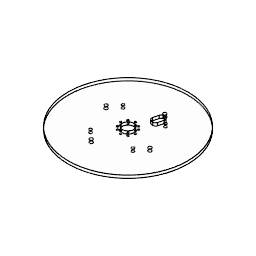
TopPlate_v60 (Autodesk Fusion 360 design; units mm, degrees)
Autodesk Fusion 360 part; units mm, degrees
note: some values were not read from the file. Set by a fixed rule: which face or edge a step refers to.
derive "Sketch1" from "ServoRail v52"
sketch "sketch 220" plane through (0, 0, 0) normal (0, 0, 1) x (1, 0, 0)
  line L0 (-23.75, 13.75) -> (23.75, 13.75) construction
  line L1 (23.75, 13.75) -> (23.75, -13.75) construction
  line L2 (23.75, -13.75) -> (-23.75, -13.75) construction
  line L3 (-23.75, -13.75) -> (-23.75, 13.75) construction
  line L4 (-23.75, 13.75) -> (23.75, -13.75) construction
  line L5 (23.75, 13.75) -> (-23.75, -13.75) construction
  line L6 (-2.75, -24.75) -> (-44.75, -24.75)
  line L7 (-44.75, -24.75) -> (-44.75, -2.75)
  line L8 (-44.75, -2.75) -> (-2.75, -2.75)
  line L9 (-2.75, -2.75) -> (-2.75, -24.75)
  line L10 (-2.75, -24.75) -> (-44.75, -2.75) construction
  line L11 (-44.75, -24.75) -> (-2.75, -2.75) construction
  line L12 (-32.75, -2.75) -> (-32.75, 4.25)
  line L13 (-32.75, 4.25) -> (-29.75, 4.25)
  line L14 (-29.75, 4.25) -> (-29.75, 0.25)
  line L15 (-26.75, 0.25) -> (-26.75, -2.75)
  line L16 (-26.75, 0.25) -> (-29.75, 0.25)
  line L17 (2.75, -44.75) -> (2.75, -2.75)
  line L18 (2.75, -32.75) -> (-4.25, -32.75)
  line L19 (-4.25, -32.75) -> (-4.25, -29.75)
  line L20 (-4.25, -29.75) -> (-0.25, -29.75)
  line L21 (-0.25, -26.75) -> (-0.25, -29.75)
  line L22 (-0.25, -26.75) -> (2.75, -26.75)
  line L23 (24.75, -44.75) -> (2.75, -44.75)
  line L24 (24.75, -2.75) -> (24.75, -44.75)
  line L25 (2.75, -2.75) -> (24.75, -2.75)
  line L26 (44.75, 2.75) -> (2.75, 2.75)
  line L27 (32.75, 2.75) -> (32.75, -4.25)
  line L28 (32.75, -4.25) -> (29.75, -4.25)
  line L29 (29.75, -4.25) -> (29.75, -0.25)
  line L30 (26.75, -0.25) -> (29.75, -0.25)
  line L31 (26.75, -0.25) -> (26.75, 2.75)
  line L32 (44.75, 24.75) -> (44.75, 2.75)
  line L33 (2.75, 24.75) -> (44.75, 24.75)
  line L34 (2.75, 2.75) -> (2.75, 24.75)
  line L35 (-2.75, 44.75) -> (-2.75, 2.75)
  line L36 (-2.75, 32.75) -> (4.25, 32.75)
  line L37 (4.25, 32.75) -> (4.25, 29.75)
  line L38 (4.25, 29.75) -> (0.25, 29.75)
  line L39 (0.25, 26.75) -> (0.25, 29.75)
  line L40 (0.25, 26.75) -> (-2.75, 26.75)
  line L41 (-24.75, 44.75) -> (-2.75, 44.75)
  line L42 (-24.75, 2.75) -> (-24.75, 44.75)
  line L43 (-2.75, 2.75) -> (-24.75, 2.75)
  line L44 (-0.25, -32.75) -> (-0.25, -35.75)
  line L45 (-0.25, -35.75) -> (-7.25, -35.75)
  line L46 (-7.25, -35.75) -> (-7.25, -26.75)
  line L47 (-7.25, -26.75) -> (-0.25, -26.75)
  line L48 (-26.75, -27.75) -> (-29.75, -27.75)
  line L49 (-29.75, -27.75) -> (-29.75, -24.75)
  line L50 (-26.75, -27.75) -> (-26.75, -31.75)
  line L51 (-26.75, -31.75) -> (-23.75, -31.75)
  line L52 (-23.75, -31.75) -> (-23.75, -24.75)
  line L53 (-29.75, -27.75) -> (-29.75, -34.75)
  line L54 (-29.75, -34.75) -> (-20.75, -34.75)
  line L55 (-20.75, -34.75) -> (-20.75, -27.75)
  line L56 (-20.75, -27.75) -> (-23.75, -27.75)
  line L57 (-20.75, -27.75) -> (-7.25, -27.75)
  line L58 (-20.75, -30.75) -> (-7.25, -30.75)
  line L59 (27.75, -29.75) -> (24.75, -29.75)
  line L60 (27.75, -29.75) -> (34.75, -29.75)
  line L61 (27.75, -26.75) -> (27.75, -29.75)
  line L62 (31.75, -23.75) -> (24.75, -23.75)
  line L63 (27.75, -26.75) -> (31.75, -26.75)
  line L64 (31.75, -26.75) -> (31.75, -23.75)
  line L65 (34.75, -29.75) -> (34.75, -20.75)
  line L66 (34.75, -20.75) -> (27.75, -20.75)
  line L67 (27.75, -20.75) -> (27.75, -23.75)
  line L68 (27.75, -20.75) -> (27.75, -7.25)
  line L69 (30.75, -20.75) -> (30.75, -7.25)
  line L70 (26.75, -7.25) -> (26.75, -0.25)
  line L71 (35.75, -7.25) -> (26.75, -7.25)
  line L72 (35.75, -0.25) -> (35.75, -7.25)
  line L73 (32.75, -0.25) -> (35.75, -0.25)
  line L74 (29.75, 27.75) -> (29.75, 24.75)
  line L75 (29.75, 27.75) -> (29.75, 34.75)
  line L76 (26.75, 27.75) -> (29.75, 27.75)
  line L77 (23.75, 31.75) -> (23.75, 24.75)
  line L78 (26.75, 27.75) -> (26.75, 31.75)
  line L79 (26.75, 31.75) -> (23.75, 31.75)
  line L80 (29.75, 34.75) -> (20.75, 34.75)
  line L81 (20.75, 34.75) -> (20.75, 27.75)
  line L82 (20.75, 27.75) -> (23.75, 27.75)
  line L83 (20.75, 27.75) -> (7.25, 27.75)
  line L84 (20.75, 30.75) -> (7.25, 30.75)
  line L85 (7.25, 26.75) -> (0.25, 26.75)
  line L86 (7.25, 35.75) -> (7.25, 26.75)
  line L87 (0.25, 35.75) -> (7.25, 35.75)
  line L88 (0.25, 32.75) -> (0.25, 35.75)
  line L89 (-27.75, 29.75) -> (-24.75, 29.75)
  line L90 (-27.75, 29.75) -> (-34.75, 29.75)
  line L91 (-27.75, 26.75) -> (-27.75, 29.75)
  line L92 (-31.75, 23.75) -> (-24.75, 23.75)
  line L93 (-27.75, 26.75) -> (-31.75, 26.75)
  line L94 (-31.75, 26.75) -> (-31.75, 23.75)
  line L95 (-34.75, 29.75) -> (-34.75, 20.75)
  line L96 (-34.75, 20.75) -> (-27.75, 20.75)
  line L97 (-27.75, 20.75) -> (-27.75, 23.75)
  line L98 (-27.75, 20.75) -> (-27.75, 7.25)
  line L99 (-30.75, 20.75) -> (-30.75, 7.25)
  line L100 (-26.75, 7.25) -> (-26.75, 0.25)
  line L101 (-35.75, 7.25) -> (-26.75, 7.25)
  line L102 (-35.75, 0.25) -> (-35.75, 7.25)
  line L103 (-32.75, 0.25) -> (-35.75, 0.25)
  circle A0 centre (0, 0) radius 56
  circle A1 centre (-41.3532, 14.4521) radius 9.125
  circle A2 centre (-14.4521, -41.3532) radius 9.125
  circle A3 centre (41.3532, -14.4521) radius 9.125
  circle A4 centre (14.4521, 41.3532) radius 9.125
  circle A5 centre (-41.3532, 14.4521) radius 11.125
  circle A6 centre (-14.4521, -41.3532) radius 11.125
  circle A7 centre (41.3532, -14.4521) radius 11.125
  circle A8 centre (14.4521, 41.3532) radius 11.125
  circle A9 centre (0, 0) radius 58
  line L104 (-41.3532, 14.4521) -> (-41.0042, 25.5716)
  line L105 (-41.3532, 14.4521) -> (-41.3532, 3.3271)
  line L106 (0, 0) -> (-41.3532, 14.4521) construction
  line L107 (-14.4521, -41.3532) -> (-25.5716, -41.0042)
  line L108 (-14.4521, -41.3532) -> (-3.3271, -41.3532)
  line L109 (41.3532, -14.4521) -> (41.0042, -25.5716)
  line L110 (41.3532, -14.4521) -> (41.3532, -3.3271)
  line L111 (14.4521, 41.3532) -> (25.5716, 41.0042)
  line L112 (14.4521, 41.3532) -> (3.3271, 41.3532)
  line L113 (2.75, 24.75) -> (-2.75, 24.75)
  line L114 (24.75, -2.75) -> (24.75, 2.75)
  line L115 (-24.75, 2.75) -> (-24.75, -2.75)
  line L116 (-2.75, -24.75) -> (2.75, -24.75)
  circle A10 centre (-7.9571, -31.4571) radius 1.75
  line L117 (-7.25, -30.75) -> (-7.9571, -31.4571)
  line L118 (-18.75, -31.75) -> (-22.75, -31.75)
  line L119 (-22.75, -31.75) -> (-22.75, -29.75)
  line L120 (-22.75, -29.75) -> (-18.75, -29.75)
  line L121 (-18.75, -29.75) -> (-18.75, -31.75)
  line L122 (-18.75, -31.75) -> (-22.75, -29.75) construction
  line L123 (-22.75, -31.75) -> (-18.75, -29.75) construction
  circle A11 centre (31.4571, -7.9571) radius 1.75
  line L124 (31.75, -22.75) -> (29.75, -22.75)
  line L125 (29.75, -22.75) -> (29.75, -18.75)
  line L126 (29.75, -18.75) -> (31.75, -18.75)
  line L127 (31.75, -18.75) -> (31.75, -22.75)
  circle A12 centre (7.9571, 31.4571) radius 1.75
  line L128 (22.75, 31.75) -> (22.75, 29.75)
  line L129 (22.75, 29.75) -> (18.75, 29.75)
  line L130 (18.75, 29.75) -> (18.75, 31.75)
  line L131 (18.75, 31.75) -> (22.75, 31.75)
  circle A13 centre (-31.4571, 7.9571) radius 1.75
  line L132 (-31.75, 22.75) -> (-29.75, 22.75)
  line L133 (-29.75, 22.75) -> (-29.75, 18.75)
  line L134 (-29.75, 18.75) -> (-31.75, 18.75)
  line L135 (-31.75, 18.75) -> (-31.75, 22.75)
  line L136 (29.75, 27.75) -> (33.8506, 28.3482) construction
  circle A14 centre (33.8506, 28.3482) radius 1.75
  circle A15 centre (-28.3482, 33.8506) radius 1.75
  circle A16 centre (-33.8506, -28.3482) radius 1.75
  circle A17 centre (28.3482, -33.8506) radius 1.75
  line L137 (-6.25, -7.75) -> (-14.25, -7.75)
  line L138 (-14.25, -7.75) -> (-14.25, -19.75)
  line L139 (-14.25, -19.75) -> (-6.25, -19.75)
  line L140 (-6.25, -19.75) -> (-6.25, -7.75)
  line L141 (-6.25, -7.75) -> (-14.25, -19.75) construction
  line L142 (-14.25, -7.75) -> (-6.25, -19.75) construction
  line L143 (19.75, -14.25) -> (19.75, -6.25)
  line L144 (7.75, -14.25) -> (19.75, -14.25)
  line L145 (19.75, -6.25) -> (7.75, -6.25)
  line L146 (7.75, -6.25) -> (7.75, -14.25)
  line L147 (14.25, 19.75) -> (6.25, 19.75)
  line L148 (14.25, 7.75) -> (14.25, 19.75)
  line L149 (6.25, 19.75) -> (6.25, 7.75)
  line L150 (6.25, 7.75) -> (14.25, 7.75)
  line L151 (-19.75, 14.25) -> (-19.75, 6.25)
  line L152 (-7.75, 14.25) -> (-19.75, 14.25)
  line L153 (-19.75, 6.25) -> (-7.75, 6.25)
  line L154 (-7.75, 6.25) -> (-7.75, 14.25)
  spline S0 degree 5 poles (-3.3271, -41.3532) (-3.3271, -42.1374) (-3.2169, -43.6541) (-2.7212, -45.7746) (-1.5233, -48.3293) (0.3412, -51.1793) (1.6763, -53.2302) (2.3663, -54.6364) (2.6513, -55.5109) (2.75, -55.9324) knots 0 0 0 0 0 0 0.2 0.4 0.6 0.8 1 1 1 1 1 1
  line L155 (-3.3271, -39.4276) -> (-3.3271, -43.2787)
  line L156 (2.5, -54.8649) -> (3, -57)
  line L157 (2.75, -44.75) -> (2.75, -55.9324) construction
  spline S1 degree 3 poles (-5.3271, -41.3532) (-5.3271, -43.6244) (-4.7917, -45.7291) (-3.9986, -47.5464) (-3.0648, -49.6861) (-1.8311, -51.476) (-0.8806, -52.9928) (-0.0937, -54.2485) (0.4782, -55.3083) (0.7178, -56.0783) (0.7516, -56.1872) (0.7797, -56.2904) (0.8027, -56.3885) knots 0 0 0 0 0.303965 0.303965 0.303965 0.661847 0.661847 0.661847 0.958125 0.958125 0.958125 1 1 1 1
  line L158 (0.6913, -55.9957) -> (2.75, -55.9324)
  spline S2 degree 5 poles (41.3532, -3.3271) (42.1374, -3.3271) (43.6541, -3.2169) (45.7746, -2.7212) (48.3293, -1.5233) (51.1793, 0.3412) (53.2302, 1.6763) (54.6364, 2.3663) (55.5109, 2.6513) (55.9324, 2.75) knots 0 0 0 0 0 0 0.2 0.4 0.6 0.8 1 1 1 1 1 1
  spline S3 degree 3 poles (41.3532, -5.3271) (43.6244, -5.3271) (45.7291, -4.7917) (47.5464, -3.9986) (49.6861, -3.0648) (51.476, -1.8311) (52.9928, -0.8806) (54.2485, -0.0937) (55.3083, 0.4782) (56.0783, 0.7178) (56.1872, 0.7516) (56.2904, 0.7797) (56.3885, 0.8027) knots 0 0 0 0 0.303965 0.303965 0.303965 0.661847 0.661847 0.661847 0.958125 0.958125 0.958125 1 1 1 1
  line L159 (55.9957, 0.6913) -> (55.9324, 2.75)
  spline S4 degree 5 poles (3.3271, 41.3532) (3.3271, 42.1374) (3.2169, 43.6541) (2.7212, 45.7746) (1.5233, 48.3293) (-0.3412, 51.1793) (-1.6763, 53.2302) (-2.3663, 54.6364) (-2.6513, 55.5109) (-2.75, 55.9324) knots 0 0 0 0 0 0 0.2 0.4 0.6 0.8 1 1 1 1 1 1
  spline S5 degree 3 poles (5.3271, 41.3532) (5.3271, 43.6244) (4.7917, 45.7291) (3.9986, 47.5464) (3.0648, 49.6861) (1.8311, 51.476) (0.8806, 52.9928) (0.0937, 54.2485) (-0.4782, 55.3083) (-0.7178, 56.0783) (-0.7516, 56.1872) (-0.7797, 56.2904) (-0.8027, 56.3885) knots 0 0 0 0 0.303965 0.303965 0.303965 0.661847 0.661847 0.661847 0.958125 0.958125 0.958125 1 1 1 1
  line L160 (-0.6913, 55.9957) -> (-2.75, 55.9324)
  spline S6 degree 5 poles (-41.3532, 3.3271) (-42.1374, 3.3271) (-43.6541, 3.2169) (-45.7746, 2.7212) (-48.3293, 1.5233) (-51.1793, -0.3412) (-53.2302, -1.6763) (-54.6364, -2.3663) (-55.5109, -2.6513) (-55.9324, -2.75) knots 0 0 0 0 0 0 0.2 0.4 0.6 0.8 1 1 1 1 1 1
  spline S7 degree 3 poles (-41.3532, 5.3271) (-43.6244, 5.3271) (-45.7291, 4.7917) (-47.5464, 3.9986) (-49.6861, 3.0648) (-51.476, 1.8311) (-52.9928, 0.8806) (-54.2485, 0.0937) (-55.3083, -0.4782) (-56.0783, -0.7178) (-56.1872, -0.7516) (-56.2904, -0.7797) (-56.3885, -0.8027) knots 0 0 0 0 0.303965 0.303965 0.303965 0.661847 0.661847 0.661847 0.958125 0.958125 0.958125 1 1 1 1
  line L161 (-55.9957, -0.6913) -> (-55.9324, -2.75)
  line L162 (-29.75, -34.75) -> (-37.9688, -34.75)
  line L163 (-29.75, -32.75) -> (-38, -32.75)
  spline S8 degree 5 poles (-37.9688, -34.75) (-38.3782, -34.75) (-39.1998, -34.6725) (-40.4402, -34.3239) (-42.1078, -33.4585) (-44.2076, -31.9324) (-45.8949, -30.4934) (-47.1632, -29.3318) (-48.0099, -28.5231) (-48.4336, -28.1103) knots 0 0 0 0 0 0 0.2 0.4 0.6 0.8 1 1 1 1 1 1
  line L164 (-37, -34.75) -> (-38.9375, -34.75)
  spline S9 degree 3 poles (-37.9688, -32.75) (-38.6389, -32.75) (-39.3828, -32.5469) (-40.2776, -32.0885) (-41.7597, -31.3293) (-43.513, -29.9305) (-45.2704, -28.34) (-45.8565, -27.8096) (-46.4464, -27.2542) (-47.0377, -26.678) knots 0 0 0 0 0.31167 0.31167 0.31167 0.827845 0.827845 0.827845 1 1 1 1
  line L165 (-48.4336, -28.1103) -> (-47.0377, -26.678)
  line L166 (34.75, -29.75) -> (34.75, -37.9688)
  line L167 (32.75, -29.75) -> (32.75, -38)
  spline S10 degree 3 poles (32.75, -37.9688) (32.75, -38.6389) (32.5469, -39.3828) (32.0885, -40.2776) (31.3293, -41.7597) (29.9305, -43.513) (28.34, -45.2704) (27.8096, -45.8565) (27.2542, -46.4464) (26.678, -47.0377) knots 0 0 0 0 0.31167 0.31167 0.31167 0.827845 0.827845 0.827845 1 1 1 1
  spline S11 degree 5 poles (34.75, -37.9688) (34.75, -38.3782) (34.6725, -39.1998) (34.3239, -40.4402) (33.4585, -42.1078) (31.9324, -44.2076) (30.4934, -45.8949) (29.3318, -47.1632) (28.5231, -48.0099) (28.1103, -48.4336) knots 0 0 0 0 0 0 0.2 0.4 0.6 0.8 1 1 1 1 1 1
  line L168 (28.1103, -48.4336) -> (26.678, -47.0377)
  line L169 (29.75, 34.75) -> (37.9688, 34.75)
  line L170 (29.75, 32.75) -> (38, 32.75)
  spline S12 degree 3 poles (37.9688, 32.75) (38.6389, 32.75) (39.3828, 32.5469) (40.2776, 32.0885) (41.7597, 31.3293) (43.513, 29.9305) (45.2704, 28.34) (45.8565, 27.8096) (46.4464, 27.2542) (47.0377, 26.678) knots 0 0 0 0 0.31167 0.31167 0.31167 0.827845 0.827845 0.827845 1 1 1 1
  spline S13 degree 5 poles (37.9688, 34.75) (38.3782, 34.75) (39.1998, 34.6725) (40.4402, 34.3239) (42.1078, 33.4585) (44.2076, 31.9324) (45.8949, 30.4934) (47.1632, 29.3318) (48.0099, 28.5231) (48.4336, 28.1103) knots 0 0 0 0 0 0 0.2 0.4 0.6 0.8 1 1 1 1 1 1
  line L171 (48.4336, 28.1103) -> (47.0377, 26.678)
  line L172 (-34.75, 29.75) -> (-34.75, 37.9688)
  line L173 (-32.75, 29.75) -> (-32.75, 38)
  spline S14 degree 3 poles (-32.75, 37.9688) (-32.75, 38.6389) (-32.5469, 39.3828) (-32.0885, 40.2776) (-31.3293, 41.7597) (-29.9305, 43.513) (-28.34, 45.2704) (-27.8096, 45.8565) (-27.2542, 46.4464) (-26.678, 47.0377) knots 0 0 0 0 0.31167 0.31167 0.31167 0.827845 0.827845 0.827845 1 1 1 1
  spline S15 degree 5 poles (-34.75, 37.9688) (-34.75, 38.3782) (-34.6725, 39.1998) (-34.3239, 40.4402) (-33.4585, 42.1078) (-31.9324, 44.2076) (-30.4934, 45.8949) (-29.3318, 47.1632) (-28.5231, 48.0099) (-28.1103, 48.4336) knots 0 0 0 0 0 0 0.2 0.4 0.6 0.8 1 1 1 1 1 1
  line L174 (-28.1103, 48.4336) -> (-26.678, 47.0377)
  point P0 (-23.75, -13.75)
  point P1 (-20.75, -30.75)
  point P2 (-10.25, -13.75)
extrude "Extrude1" add sketch "sketch 220" along normal blind 3 contours L6 L17 L22 L46 L47 L52 L56 L57 L116 | L6 L7 L8 L9 | L8 L9 L17 L25 L26 L34 L35 L43 L113 L114 L115 L116 | L6 L48 L49 L50 L51 L52 | L17 L23 L24 L25 | L6 L7 L8 L12 L49 L53 L102 L103 A0 A5 S6 L163 S9 L165 | L48 L50 L51 L52 L53 L54 L55 L56 A6 L118 L119 L120 | L8 L15 L42 L92 L97 L98 L100 L101 L115 | L17 L18 L19 L20 L21 L22 | L46 L55 L57 L58 A6 A10 L120 L121 | L8 L12 L13 L14 L15 L16 | L35 L41 L42 L43 | L17 L18 L23 L24 L44 L45 L59 L60 A0 A6 S0 L167 S10 L168 | L18 L19 L20 L21 L44 L45 L46 L47 A6 A10 | L24 L26 L31 L62 L67 L68 L70 L71 L114 | L53 L162 L163 S8 L164 S9 L165 | L55 L58 L120 L121 | L55 L118 L119 L120 | L12 L13 L14 L16 L100 L101 L102 L103 A5 A13 | L42 L89 L91 L92 L93 L94 | L24 L59 L61 L62 L63 L64 | L26 L32 L33 L34 | L54 A0 A6 S1 L162 S8 L164 | L55 L58 A6 L118 L121 | L35 L36 L41 L42 L87 L88 L89 L90 A0 A8 S4 L173 S14 L174 | L90 L91 L92 L93 L94 L95 L96 L97 A5 L132 L133 L135 | L33 L35 L40 L77 L82 L83 L85 L86 L113 | L60 L61 L62 L63 L64 L65 L66 L67 A7 L124 L125 L127 | L26 L27 L28 L29 L30 L31 | L54 L55 A6 | L54 A2 A6 L107 | L55 A6 L118 | L58 A6 L121 | L58 A6 A10 | L96 L98 L99 L101 A5 A13 L133 L134 | L35 L36 L37 L38 L39 L40 | L45 A2 A6 L108 | L45 L46 A6 A10 | L66 L68 L69 L71 A7 A11 L125 L126 | L26 L27 L32 L33 L72 L73 L74 L75 A0 A7 S2 L170 S12 L171 | L27 L28 L29 L30 L70 L71 L72 L73 A7 A11 | L46 L55 L58 A2 A6 A10 L118 L121 | A2 L107 L108 | A2 A6 L107 S1 | A6 L118 L121 | L58 A6 | L102 A1 A5 L105 | L101 L102 A5 A13 | L90 L172 L173 S14 S15 L174 | L96 L99 L133 L134 | L96 L132 L133 L135 | L36 L37 L38 L39 L85 L86 L87 L88 A8 A12 | L33 L74 L76 L77 L78 L79 | A6 S0 S1 L158 | A6 L108 S1 | L60 L166 L167 S10 S11 L168 | L66 L69 L125 L126 | L66 L124 L125 L127 | A2 L107 L108 | L96 L99 L101 A1 A5 A13 L134 L135 | A1 L104 L105 | A5 S6 S7 L161 | A5 L105 S7 | L95 A0 A5 S7 L172 S15 | L96 L99 A5 L134 L135 | L75 L76 L77 L78 L79 L80 L81 L82 A8 L128 L129 L131 | A0 L158 | L65 A0 A7 S3 L166 S11 | L66 L69 A7 L126 L127 | A0 L161 | A1 A5 L104 S7 | A1 L104 L105 | L99 A5 A13 | L95 L96 A5 | L95 A1 A5 L104 | L96 A5 L135 | L99 A5 L134 | L81 L83 L84 L86 A8 A12 L129 L130 | L65 L66 A7 | L65 A3 A7 L109 | L66 A7 L127 | L69 A7 L126 | L71 L72 A7 A11 | L69 A7 A11 | L72 A3 A7 L110 | L99 A5 | A5 L134 L135 | L87 A4 A8 L112 | L86 L87 A8 A12 | L75 L169 L170 S12 S13 L171 | L81 L84 L129 L130 | L81 L128 L129 L131 | L66 L69 L71 A3 A7 A11 L126 L127 | A3 L109 L110 | A3 A7 L109 S3 | A7 L126 L127 | L69 A7 | A7 S2 S3 L159 | A7 L110 S3 | A8 S4 S5 L160 | A0 L160 | L81 L84 L86 A4 A8 A12 L130 L131 | A4 L111 L112 | A8 L112 S5 | L84 A8 A12 | L80 A0 A8 S5 L169 S13 | L81 L84 A8 L130 L131 | A0 L159 | A3 L109 L110 | A4 A8 L111 S5 | A4 L111 L112 | L80 A4 A8 L111 | L80 L81 A8 | L84 A8 | L81 A8 L131 | L84 A8 L130 | A8 L130 L131 | A14 | A15 | A16 | A17 | L137 L138 L139 L140 | L143 L144 L145 L146 | L147 L148 L149 L150 | L151 L152 L153 L154
move_face "OffsetFaces5" offset 8 5 faces at (55.9987, 0.3841, 2) (55.9924, 0.9202, 1) (-2.5214, 55.9432, 2) (-55.9432, -2.5214, 2) (2.5214, -55.9432, 2)
sketch "Sketch1" plane through (0, 0, 3) normal (0, 0, 1) x (-1, 0, 0)
  circle A0 centre (-7, 47.5) radius 2
  circle A1 centre (-20, 47.5) radius 2
  line L0 (-20, 47.5) -> (-7, 47.5) construction
  circle A2 centre (0, 0) radius 6
  line L1 (0, 0) -> (-13.5, 47.5) construction
  circle A3 centre (-47.5, -20) radius 2
  circle A4 centre (-47.5, -7) radius 2
  circle A5 centre (20, -47.5) radius 2
  circle A6 centre (7, -47.5) radius 2
  circle A7 centre (47.5, 20) radius 2
  circle A8 centre (47.5, 7) radius 2
  circle A9 centre (22.7166, -17.3624) radius 1.5
  line L2 (22.7166, -17.3624) -> (7.7166, -17.3624) construction
  circle A10 centre (7.7166, -17.3624) radius 1.75
  line L3 (0, 0) -> (7.7166, -17.3624) construction
  circle A11 centre (17.3624, 22.7166) radius 1.5
  circle A12 centre (17.3624, 7.7166) radius 1.75
  circle A13 centre (-22.7166, 17.3624) radius 1.5
  circle A14 centre (-7.7166, 17.3624) radius 1.75
  circle A15 centre (-17.3624, -22.7166) radius 1.5
  circle A16 centre (-17.3624, -7.7166) radius 1.75
  circle A17 centre (0, 0) radius 64
  line L4 (0, 0) -> (8, 0) construction
  circle A18 centre (8, 0) radius 1
  circle A19 centre (5.6569, 5.6569) radius 1
  circle A20 centre (0, 8) radius 1
  circle A21 centre (-5.6569, 5.6569) radius 1
  circle A22 centre (-8, 0) radius 1
  circle A23 centre (-5.6569, -5.6569) radius 1
  circle A24 centre (0, -8) radius 1
  circle A25 centre (5.6569, -5.6569) radius 1
  line L5 (6, 0) -> (8, 0)
  circle A26 centre (0, 0) radius 11.5
  line L6 (0, -8) -> (0, -6) construction
  line L7 (0.15, -6.5021) -> (-0.15, -6.5021) construction
  line L8 (-0.15, -6.5021) -> (-0.15, -7.0113)
  line L9 (0.15, -6.5021) -> (0.15, -7.0113)
  line L10 (0.15, -6.5021) -> (0.15, -5.9981)
  line L11 (-0.15, -6.5021) -> (-0.15, -5.9981)
  line L12 (4.7037, -4.4916) -> (5.0638, -4.8517)
  line L13 (4.4916, -4.7037) -> (4.8517, -5.0638)
  line L14 (4.4916, -4.7037) -> (4.1352, -4.3474)
  line L15 (4.7037, -4.4916) -> (4.3474, -4.1352)
  line L16 (6.5021, 0.15) -> (7.0113, 0.15)
  line L17 (6.5021, -0.15) -> (7.0113, -0.15)
  line L18 (6.5021, -0.15) -> (5.9981, -0.15)
  line L19 (6.5021, 0.15) -> (5.9981, 0.15)
  line L20 (4.4916, 4.7037) -> (4.8517, 5.0638)
  line L21 (4.7037, 4.4916) -> (5.0638, 4.8517)
  line L22 (4.7037, 4.4916) -> (4.3474, 4.1352)
  line L23 (4.4916, 4.7037) -> (4.1352, 4.3474)
  line L24 (-0.15, 6.5021) -> (-0.15, 7.0113)
  line L25 (0.15, 6.5021) -> (0.15, 7.0113)
  line L26 (0.15, 6.5021) -> (0.15, 5.9981)
  line L27 (-0.15, 6.5021) -> (-0.15, 5.9981)
  line L28 (-4.7037, 4.4916) -> (-5.0638, 4.8517)
  line L29 (-4.4916, 4.7037) -> (-4.8517, 5.0638)
  line L30 (-4.4916, 4.7037) -> (-4.1352, 4.3474)
  line L31 (-4.7037, 4.4916) -> (-4.3474, 4.1352)
  line L32 (-6.5021, -0.15) -> (-7.0113, -0.15)
  line L33 (-6.5021, 0.15) -> (-7.0113, 0.15)
  line L34 (-6.5021, 0.15) -> (-5.9981, 0.15)
  line L35 (-6.5021, -0.15) -> (-5.9981, -0.15)
  line L36 (-4.4916, -4.7037) -> (-4.8517, -5.0638)
  line L37 (-4.7037, -4.4916) -> (-5.0638, -4.8517)
  line L38 (-4.7037, -4.4916) -> (-4.3474, -4.1352)
  line L39 (-4.4916, -4.7037) -> (-4.1352, -4.3474)
  circle A27 centre (3.8268, 9.2388) radius 1.5
  line L40 (5.6569, 5.6569) -> (0, 8) construction
  line L41 (2.8284, 6.8284) -> (3.8268, 9.2388) construction
  circle A28 centre (-9.2388, 3.8268) radius 1.5
  circle A29 centre (-3.8268, -9.2388) radius 1.5
  circle A30 centre (9.2388, -3.8268) radius 1.5
  line L42 (3.8268, 9.2388) -> (9.3731, 23.1758) construction
  circle A31 centre (9.3731, 23.1758) radius 6
  circle A32 centre (-23.1758, 9.3731) radius 6
  circle A33 centre (-9.3731, -23.1758) radius 6
  circle A34 centre (23.1758, -9.3731) radius 6
  line L43 (9.3731, 23.1758) -> (16.4577, 40.9201) construction
  line L44 (15.4708, 31.706) -> (10.8272, 33.56)
  line L45 (9.9003, 31.2382) -> (11.7542, 35.8818)
  line L46 (9.9003, 31.2382) -> (11.7542, 35.8818)
  line L47 (11.7542, 35.8818) -> (9.8968, 36.6234)
  line L48 (9.8968, 36.6234) -> (8.0428, 31.9798)
  line L49 (8.0428, 31.9798) -> (9.9003, 31.2382)
  line L50 (16.4012, 28.6426) -> (14.5438, 29.3842)
  line L51 (18.2552, 33.2862) -> (16.4012, 28.6426)
  line L52 (14.5438, 29.3842) -> (16.3978, 34.0278)
  line L53 (16.3978, 34.0278) -> (18.2552, 33.2862)
  line L54 (-31.9798, 8.0428) -> (-31.2382, 9.9003)
  line L55 (-31.2382, 9.9003) -> (-35.8818, 11.7542)
  line L56 (-35.8818, 11.7542) -> (-36.6234, 9.8968)
  line L57 (-36.6234, 9.8968) -> (-31.9798, 8.0428)
  line L58 (-29.3842, 14.5438) -> (-34.0278, 16.3978)
  line L59 (-28.6426, 16.4012) -> (-29.3842, 14.5438)
  line L60 (-33.2862, 18.2552) -> (-28.6426, 16.4012)
  line L61 (-34.0278, 16.3978) -> (-33.2862, 18.2552)
  line L62 (-8.0428, -31.9798) -> (-9.9003, -31.2382)
  line L63 (-9.9003, -31.2382) -> (-11.7542, -35.8818)
  line L64 (-11.7542, -35.8818) -> (-9.8968, -36.6234)
  line L65 (-9.8968, -36.6234) -> (-8.0428, -31.9798)
  line L66 (-14.5438, -29.3842) -> (-16.3978, -34.0278)
  line L67 (-16.4012, -28.6426) -> (-14.5438, -29.3842)
  line L68 (-18.2552, -33.2862) -> (-16.4012, -28.6426)
  line L69 (-16.3978, -34.0278) -> (-18.2552, -33.2862)
  line L70 (31.9798, -8.0428) -> (31.2382, -9.9003)
  line L71 (31.2382, -9.9003) -> (35.8818, -11.7542)
  line L72 (35.8818, -11.7542) -> (36.6234, -9.8968)
  line L73 (36.6234, -9.8968) -> (31.9798, -8.0428)
  line L74 (29.3842, -14.5438) -> (34.0278, -16.3978)
  line L75 (28.6426, -16.4012) -> (29.3842, -14.5438)
  line L76 (33.2862, -18.2552) -> (28.6426, -16.4012)
  line L77 (34.0278, -16.3978) -> (33.2862, -18.2552)
  line L78 (-14.2076, -26.7294) -> (-11.8649, -17.7176)
  line L79 (-6.8814, -28.6339) -> (-4.5387, -19.6221)
  line L80 (-9.3731, -23.1758) -> (-10.8827, -28.9827)
  circle A35 centre (-7.9571, -31.4571) radius 1.75
  circle A36 centre (7.9571, 31.4571) radius 1.75
  circle A37 centre (31.4571, -7.9571) radius 1.75
  circle A38 centre (-31.4571, 7.9571) radius 1.75
  point P0 (0, -6.5021)
  point P1 (13.149, 32.633)
  dimension "d3" = 4
  dimension "d4" = 4
  dimension "d5" = 13
  dimension "d7" = 47.5
  dimension "d8" = 13.5
  dimension "d10" = 360
  dimension "d20" = 3
  dimension "d21" = 15
  dimension "d22" = 3.5
  dimension "d23" = 19
  dimension "d24" = 113.962
  dimension "d25" = 2
  dimension "d28" = 360
  dimension "d30" = 2
  dimension "d33" = 12
  dimension "d34" = 23
  dimension "d35" = 0.3
  dimension "d40" = 3
  dimension "d42" = 360
  dimension "d43" = 12
  dimension "d44" = 15
  dimension "d45" = 5
  dimension "d46" = 5
  dimension "d47" = 2
  constraint coincident A1.centre L0.start
  constraint coincident A0.centre L0.end
  constraint horizontal L0
  constraint coincident A2.centre L1.start
  constraint midpoint L0 L1.end
  constraint coincident A9.centre L2.start
  constraint horizontal L2
  constraint coincident L2.end A10.centre
  constraint horizontal L4
  constraint coincident L4.end A18.centre
  constraint coincident L4 L5.start
  constraint coincident A2 L5.start
  constraint concentric A2 A26
  constraint coincident A24.centre L6.start
  constraint coincident A2 L6.end
  constraint vertical L6
  constraint midpoint L7 P0
  constraint coincident L6 P0
  constraint perpendicular L6 L7
  constraint coincident A24 L8.end
  constraint perpendicular L7 L8
  constraint coincident A24 L9.end
  constraint perpendicular L7 L9
  constraint coincident A2 L10.end
  constraint perpendicular L7 L10
  constraint coincident A2 L11.end
  constraint perpendicular L7 L11
  constraint tangent A26 A27
  constraint coincident A19.centre L40.start
  constraint coincident A20.centre L40.end
  constraint midpoint L40 L41.start
  constraint coincident A27.centre L41.end
  constraint perpendicular L40 L41
  constraint coincident L42.end A31.centre
  constraint midpoint L44 P1
  constraint coincident L43 P1
  constraint perpendicular L43 L44
  constraint midpoint L44.end L45
  constraint perpendicular L44 L45
  constraint perpendicular L46 L47
  constraint parallel L46 L48
  constraint parallel L47 L49
  constraint symmetric L43 L45.start L50.end
  constraint symmetric L43 L45.end L52.end
  constraint symmetric L43 L47.end L51.start
  constraint symmetric L43 L48.end L50.start
  constraint coincident A33 L78.start
  constraint coincident A33 L78.end
  constraint coincident A33 L79.start
  constraint coincident A33 L79.end
  constraint parallel L78 L79
  constraint coincident A33.centre L80.start
  constraint coincident A33 L80.end
  constraint parallel L78 L80
  constraint symmetric L78 L79 L80
  measures "d3" diameter of A0
  measures "d4" diameter of A1
  measures "d5" distance of A1.centre A0.centre
  measures "d7" vertical distance of A2.centre L1.end
  measures "d8" horizontal distance of A2.centre L1.end
  measures "d20" diameter of A9
  measures "d21" distance of A9.centre L2.end
  measures "d22" diameter of A10
  measures "d23" distance of L2.end A2.centre
  measures "d24" angle of L2 L3
  measures "d25" diameter of A18
  measures "d30" distance of L4.end L5.start
  measures "d33" diameter of A2
  measures "d34" diameter of A26
  measures "d35" distance of L7.start L7.end
  measures "d40" diameter of A27
  measures "d43" diameter of A31
  measures "d44" distance of A27.centre L42.end
  measures "d45" distance of L44.start L44.end
  measures "d46" distance of L45.start L45.end
  measures "d47" distance of L45.start L48.end
extrude "Extrude2" cut sketch "Sketch1" against normal blind 25 contours A2 | A18 | A19 | A25 | A20 | A24 | A21 | A23 | A22 | A9 | A11 | A13 | A15 | A33 L78 L79
derive "ExternalDerived2" from "OuterShellUpper v68"
sketch "Sketch4" plane through (0, 0, 3) normal (0, 0, 1) x (-1, 0, 0)
  circle A0 centre (5.6569, -5.6569) radius 1
  circle A1 centre (0, -8) radius 1
  circle A2 centre (-17.3624, -22.7166) radius 1.5
  circle A3 centre (17.3624, 22.7166) radius 1.5
  circle A4 centre (-5.6569, -5.6569) radius 1
  circle A5 centre (-5.6569, 5.6569) radius 1
  circle A6 centre (0, 8) radius 1
  circle A7 centre (5.6569, 5.6569) radius 1
  circle A8 centre (0, 0) radius 6
  circle A9 centre (-22.7166, 17.3624) radius 1.5
  circle A10 centre (22.7166, -17.3624) radius 1.5
  circle A11 centre (-8, 0) radius 1
  circle A12 centre (8, 0) radius 1
  circle A13 centre (6.0806, -14.2339) radius 1.5
  circle A14 centre (2, -15.5) radius 1
  circle A15 centre (14.2339, 6.0806) radius 1.5
  circle A16 centre (15.5, 2) radius 1
  circle A17 centre (-6.0806, 14.2339) radius 1.5
  circle A18 centre (-2, 15.5) radius 1
  circle A19 centre (-14.2339, -6.0806) radius 1.5
  circle A20 centre (-15.5, -2) radius 1
  circle A21 centre (0, 0) radius 64
  line L0 (-4.5387, -19.6221) -> (-6.8814, -28.6339)
  arc A22 (-14.2076, -26.7294) -> (-6.8814, -28.6339) centre (-9.3731, -23.1758) ccw
  line L1 (-14.2076, -26.7294) -> (-11.8649, -17.7176)
  arc A23 (-4.5387, -19.6221) -> (-11.8649, -17.7176) centre (-9.3731, -23.1758) ccw
  circle A24 centre (-31.4571, 7.9571) radius 1.75
  circle A25 centre (31.4571, -7.9571) radius 1.75
  circle A26 centre (7.9571, 31.4571) radius 1.75
  circle A27 centre (-7.9571, -31.4571) radius 1.75
  dimension "d48" = 3
  dimension "d49" = 2
  dimension "d51" = 360
  measures "d48" diameter of A13
  measures "d49" diameter of A14
fillet "Fillet4" radius 3 4 edges at (6.8814, 28.6339, 1.5) (4.5387, 19.6221, 1.5) (11.8649, 17.7176, 1.5) (14.2076, 26.7294, 1.5)
sketch "Sketch7" plane through (0, 0, 3) normal (0, 0, 1) x (-1, 0, 0)
  circle A0 centre (0, 0) radius 64
  circle A1 centre (-31.4571, 7.9571) radius 1.75
  circle A2 centre (31.4571, -7.9571) radius 1.75
  circle A3 centre (7.9571, 31.4571) radius 1.75
  circle A4 centre (-7.9571, -31.4571) radius 1.75
  line L0 (-4.9815, -21.3256) -> (-6.4385, -26.9304)
  arc A5 (-9.3109, -29.1754) -> (-6.4385, -26.9304) centre (-9.342, -26.1756) ccw
  arc A6 (-12.3493, -28.3856) -> (-9.3109, -29.1754) centre (-9.3731, -23.1758) ccw
  arc A7 (-13.7647, -25.0259) -> (-12.3493, -28.3856) centre (-10.8612, -25.7807) ccw
  line L1 (-13.7647, -25.0259) -> (-12.3077, -19.4211)
  arc A8 (-9.4353, -17.1761) -> (-12.3077, -19.4211) centre (-9.4042, -20.1759) ccw
  arc A9 (-6.3969, -17.9659) -> (-9.4353, -17.1761) centre (-9.3731, -23.1758) ccw
  arc A10 (-4.9815, -21.3256) -> (-6.3969, -17.9659) centre (-7.885, -20.5708) ccw
  circle A11 centre (5.6569, -5.6569) radius 1
  circle A12 centre (0, -8) radius 1
  circle A13 centre (-17.3624, -22.7166) radius 1.5
  circle A14 centre (17.3624, 22.7166) radius 1.5
  circle A15 centre (-5.6569, -5.6569) radius 1
  circle A16 centre (-5.6569, 5.6569) radius 1
  circle A17 centre (0, 8) radius 1
  circle A18 centre (5.6569, 5.6569) radius 1
  circle A19 centre (0, 0) radius 6
  circle A20 centre (-22.7166, 17.3624) radius 1.5
  circle A21 centre (22.7166, -17.3624) radius 1.5
  circle A22 centre (-8, 0) radius 1
  circle A23 centre (8, 0) radius 1
